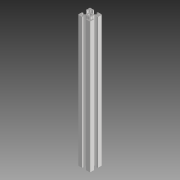
# Autodesk Inventor part: KHFS5-2020-1000
Saved by Autodesk Inventor 2020 (Build 240168000, 168)
## iProperties
Part Number: KHFS5-2020-1000
Material: Generic
Catalog Web Link: www.cadenas.de
Description: KHFS5-2020-1000-HFS5 Series Aluminum Extrusions 20,25,40mm Square -1 Slot-
Vendor: MISUMI
Document SubType Name: Modeling
Designer: partserver
Manufacturer: MISUMI
Mass: 182.243 g
Surface Area: 1734.63 cm^2
Volume: 182.243 cm^3
Density: 1 g/cm^3
Appearance: PSOLRGB-175-175-175
Category: PARTsolutions
Company: MISUMI
L: 1000
PSOL_IDENT_0: {$CADENAS_DATA\23d-libs\misumi\metric\38_al_extrusions_blackets\5\khfs5_2020_1000.prj},179 {VTYP=3D}
PSOL_IDENT_1: ,{NB=KHFS5-2020-1000},{LINA=KHFS5-2020-1000},{NN=KHFS5-2020-1000},{DATE=09.09.2019 09:03:53},{GEOMDA
PSOL_IDENT_2: TE=07.04.2011 07:47:00},{VERSION=},{LINEID=10},{WBVAR=},{WBNUMERIC=}  {NB=KHFS5-2020-1000},{LINA=KHF
PSOL_IDENT_3: S5-2020-1000},{KT=1},{PN=KHFS5-2020-1000},{TPS=KHFS5-2020},{TP=KHFS5},{FRM=2020},{TYPE=KHFS5},{MAT=A
PSOL_IDENT_4: 6N01SS-T5 Aluminum Alloy or 6005A-T5 Aluminum Alloy},{ST=Clear Anodize},{FEAT=4 Slots},{L=1000},{LTO
PSOL_IDENT_5: L=+/- 0.5},{MASS=0.50},{SA=183},{GMILX=0.742x10^4},{GMILY=0.742x10^4},{WIDTH=20},{HEIGHT=20},{TAPDEP
PSOL_IDENT_6: TH=15},{TAPSTART=0},{DRILLLENGTH=0},{DRILLDIA=4.2},{TAPPOSHOR=0},{TAPPOSVER=0},{VER=1},{DIM=1},{CLF=
PSOL_IDENT_7: HFS5-2020},{ALT3=}
NB: KHFS5-2020-1000
NN: KHFS5-2020-1000
NT: HFS5 Series Aluminum Extrusions 20,25,40mm Square -1 Slot-
NBSYN: $PN.
LINA: KHFS5-2020-1000
CATALOG: Misumi
PN: KHFS5-2020-1000
TPS: KHFS5-2020
MAT: A6N01SS-T5 Aluminum Alloy or 6005A-T5 Aluminum Alloy
ST: Clear Anodize
LTOL: +/- 0.5
SA: 183
GMILX: 0.742x10^4
GMILY: 0.742x10^4
CLF: HFS5-2020
SUPPLIER: MISUMI
ARTICLENO: KHFS5-2020-1000
BOMINFO: KHFS5-2020-1000
CREATOR: CADENAS GmbH
Title: KHFS5-2020-1000
Author: Cadenas PARTsolutions
Comments: HFS5 Series Aluminum Extrusions 20,25,40mm Square -1 Slot-
Autodesk Inventor part; units mm, degrees
sketch "Sketch_5" plane through (0, 0, 0) normal (0, 0, 1) x (1, 0, 0)
  arc A0 (-10, 3.3) -> (-9.7, 3) centre (-9.7, 3.3) ccw
  line L0 (-9.7, 3) -> (-8, 3)
  line L1 (-8, 3) -> (-8, 6)
  line L2 (-8, 6) -> (-7.0607, 6)
  line L3 (-7.0607, 6) -> (-4, 2.9393)
  line L4 (-4, 2.9393) -> (-4, 0.3)
  line L5 (-4, 0.3) -> (-3.7, 0)
  line L6 (-3.7, 0) -> (-4, -0.3)
  line L7 (-4, -0.3) -> (-4, -2.9393)
  line L8 (-4, -2.9393) -> (-7.0607, -6)
  line L9 (-7.0607, -6) -> (-8, -6)
  line L10 (-8, -6) -> (-8, -3)
  line L11 (-8, -3) -> (-9.7, -3)
  arc A1 (-9.7, -3) -> (-10, -3.3) centre (-9.7, -3.3) ccw
  line L12 (-10, -3.3) -> (-10, -9)
  arc A2 (-10, -9) -> (-9, -10) centre (-9, -9) ccw
  line L13 (-9, -10) -> (-3.3, -10)
  arc A3 (-3.3, -10) -> (-3, -9.7) centre (-3.3, -9.7) ccw
  line L14 (-3, -9.7) -> (-3, -8)
  line L15 (-3, -8) -> (-6, -8)
  line L16 (-6, -8) -> (-6, -7.0607)
  line L17 (-6, -7.0607) -> (-2.9393, -4)
  line L18 (-2.9393, -4) -> (-0.3, -4)
  line L19 (-0.3, -4) -> (0, -3.7)
  line L20 (0, -3.7) -> (0.3, -4)
  line L21 (0.3, -4) -> (2.9393, -4)
  line L22 (2.9393, -4) -> (6, -7.0607)
  line L23 (6, -7.0607) -> (6, -8)
  line L24 (6, -8) -> (3, -8)
  line L25 (3, -8) -> (3, -9.7)
  arc A4 (3, -9.7) -> (3.3, -10) centre (3.3, -9.7) ccw
  line L26 (3.3, -10) -> (9, -10)
  arc A5 (9, -10) -> (10, -9) centre (9, -9) ccw
  line L27 (10, -9) -> (10, -3.3)
  arc A6 (10, -3.3) -> (9.7, -3) centre (9.7, -3.3) ccw
  line L28 (9.7, -3) -> (8, -3)
  line L29 (8, -3) -> (8, -6)
  line L30 (8, -6) -> (7.0607, -6)
  line L31 (7.0607, -6) -> (4, -2.9393)
  line L32 (4, -2.9393) -> (4, -0.3)
  line L33 (4, -0.3) -> (3.7, 0)
  line L34 (3.7, 0) -> (4, 0.3)
  line L35 (4, 0.3) -> (4, 2.9393)
  line L36 (4, 2.9393) -> (7.0607, 6)
  line L37 (7.0607, 6) -> (8, 6)
  line L38 (8, 6) -> (8, 3)
  line L39 (8, 3) -> (9.7, 3)
  arc A7 (9.7, 3) -> (10, 3.3) centre (9.7, 3.3) ccw
  line L40 (10, 3.3) -> (10, 9)
  arc A8 (10, 9) -> (9, 10) centre (9, 9) ccw
  line L41 (9, 10) -> (3.3, 10)
  arc A9 (3.3, 10) -> (3, 9.7) centre (3.3, 9.7) ccw
  line L42 (3, 9.7) -> (3, 8)
  line L43 (3, 8) -> (6, 8)
  line L44 (6, 8) -> (6, 7.0607)
  line L45 (6, 7.0607) -> (2.9393, 4)
  line L46 (2.9393, 4) -> (0.3, 4)
  line L47 (0.3, 4) -> (0, 3.7)
  line L48 (0, 3.7) -> (-0.3, 4)
  line L49 (-0.3, 4) -> (-2.9393, 4)
  line L50 (-2.9393, 4) -> (-6, 7.0607)
  line L51 (-6, 7.0607) -> (-6, 8)
  line L52 (-6, 8) -> (-3, 8)
  line L53 (-3, 8) -> (-3, 9.7)
  arc A10 (-3, 9.7) -> (-3.3, 10) centre (-3.3, 9.7) ccw
  line L54 (-3.3, 10) -> (-9, 10)
  arc A11 (-9, 10) -> (-10, 9) centre (-9, 9) ccw
  line L55 (-10, 9) -> (-10, 3.3)
  circle A12 centre (0, 0) radius 2.1
  constraints: 112 end point, 24 point on circle, 13 centre point
extrude "Extrusion1" add sketch "Sketch_5" against normal blind 1000
ref_plane "to_frame_XY" through (0, 0, 0) normal (0, 0, 1) x (1, 0, 0)
ref_plane "to_frame_YZ" through (0, 0, 0) normal (1, 0, 0) x (0, 1, 0)
ref_plane "to_frame_ZX" through (0, 0, 0) normal (0, 1, 0) x (0, 0, 1)
sketch "Sketch2" plane through (-10, -3.3, -1000) normal (-1, 0, 0) x (0, 0, 1)
  line L0 (-212.6604, -150.7885) -> (785, -150.7885)
  line L1 (785, -150.7885) -> (785, 147.9074)
  line L2 (785, 147.9074) -> (-212.6604, 147.9074)
  line L3 (-212.6604, 147.9074) -> (-212.6604, -150.7885)
  point P0 (1000, 3.3)
  dimension "d3" = 215
  constraints: 8 end point, 2 parallel, 1 horizontal, 1 perpendicular
  measures "d3" distance from line of point (1000, 3.3) L1
extrude "Extrusion2" cut sketch "Sketch2" against normal through all
equation "\"d0\" = L"
equation "\"L\" = 1000"
body "Solid1"
